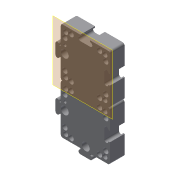
# Autodesk Inventor part: 30_cellSTORM_UC2_motorized_xystage_coupler_fiberlauncher
Saved by Autodesk Inventor 2022 (Build 260153000, 153)
## iProperties
Created: 2021-10-28
Part Number: 30_cellSTORM_UC2_motorized_xystage_coupler_fiberlauncher
Material: Generic
Document SubType Name: Modeling
Designer: diederichbenedict
Density: 1 g/cm^3
Appearance: Default
Author: diederichbenedict
Autodesk Inventor part; units mm, degrees
ref_plane "YZ Plane" through (0, 0, 0) normal (1, 0, 0) x (0, 1, 0)
ref_plane "XZ Plane" through (0, 0, 0) normal (0, 1, 0) x (-1, 0, 0)
ref_plane "XY Plane" through (0, 0, 0) normal (0, 0, 1) x (1, 0, 0)
ref_plane "Work Plane1" through (0, 100, 0) normal (0, 0, 1) x (1, 0, 0)
sketch "Sketch1" plane through (0, 100, 0) normal (0, 0, 1) x (1, 0, 0)
  circle A0 centre (-5.5948, 23.1279) radius 1.5 projected
  line L0 (30.2052, 32.2052) -> (0.2052, 32.2052) projected
  arc A1 (32.2052, 30.2052) -> (30.2052, 32.2052) centre (30.2052, 30.2052) ccw projected
  line L1 (32.2052, 30.2052) -> (32.2052, 0.2052) projected
  arc A2 (30.2052, -1.7948) -> (32.2052, 0.2052) centre (30.2052, 0.2052) ccw projected
  line L2 (15.6052, -1.7948) -> (30.2052, -1.7948) projected
  circle A3 centre (15.6052, -5.7948) radius 4 projected
  line L3 (0.2052, -1.7948) -> (15.6052, -1.7948) projected
  arc A4 (-1.7948, 0.2052) -> (0.2052, -1.7948) centre (0.2052, 0.2052) ccw projected
  line L4 (-1.7948, 0.2052) -> (-1.7948, 15.4052) projected
  circle A5 centre (-5.7948, 15.4052) radius 4 projected
  line L5 (-1.7948, 15.4052) -> (-1.7948, 30.2052) projected
  arc A6 (0.2052, 32.2052) -> (-1.7948, 30.2052) centre (0.2052, 30.2052) ccw projected
  circle A7 centre (-4.7948, -4.7948) radius 2.425 projected
  circle A8 centre (0.7052, -5.5948) radius 2.65 projected
  circle A9 centre (-5.5948, 0.7052) radius 2.65 projected
  circle A10 centre (-5.5948, 29.7052) radius 2.65 projected
  circle A11 centre (0.7052, 36.0052) radius 2.65 projected
  circle A12 centre (-4.7948, 35.2052) radius 2.425 projected
  circle A13 centre (36.0052, 0.7052) radius 2.65 projected
  circle A14 centre (29.7052, -5.5948) radius 2.65 projected
  circle A15 centre (35.2052, -4.7948) radius 2.425 projected
  circle A16 centre (36.0052, 29.7052) radius 2.65 projected
  circle A17 centre (29.7052, 36.0052) radius 2.65 projected
  circle A18 centre (35.2052, 35.2052) radius 2.425 projected
  line L6 (20.0856, 40.2052) -> (20.0856, 39.0762) projected
  arc A19 (20.0856, 39.0762) -> (20.4256, 38.6775) centre (20.4974, 39.083) ccw projected
  line L7 (20.4256, 38.6775) -> (20.5462, 38.647) projected
  arc A20 (20.0038, 34.5391) -> (20.5462, 38.647) centre (20.2052, 36.6023) ccw projected
  line L8 (20.0038, 34.5391) -> (10.2052, 34.5391) projected
  arc A21 (9.7873, 38.6768) -> (10.2052, 34.5391) centre (10.2052, 36.6291) ccw projected
  arc A22 (9.7873, 38.6768) -> (10.1151, 39.0783) centre (9.7054, 39.0783) ccw projected
  line L9 (10.1151, 39.0783) -> (10.1151, 40.2052) projected
  line L10 (10.1151, 40.2052) -> (-7.7948, 40.2052) projected
  arc A23 (-7.7948, 40.2052) -> (-9.7948, 38.2052) centre (-7.7948, 38.2052) ccw projected
  line L11 (-9.7948, 20.2052) -> (-9.7948, 38.2052) projected
  line L12 (-10.8453, 20.2052) -> (-9.7948, 20.2052) projected
  arc A24 (-11.3352, 20.6052) -> (-10.8453, 20.2052) centre (-10.8453, 20.7052) ccw projected
  arc A25 (-11.3352, 20.6052) -> (-15.2948, 20.2052) centre (-13.2948, 20.2052) ccw projected
  line L13 (-15.2948, 10.2052) -> (-15.2948, 20.2052) projected
  arc A26 (-15.2948, 10.2052) -> (-11.3352, 9.8052) centre (-13.2948, 10.2052) ccw projected
  arc A27 (-10.8453, 10.2052) -> (-11.3352, 9.8052) centre (-10.8453, 9.7052) ccw projected
  line L14 (-9.7948, 10.2052) -> (-10.8453, 10.2052) projected
  line L15 (-9.7948, -7.7948) -> (-9.7948, 10.2052) projected
  arc A28 (-9.7948, -7.7948) -> (-7.7948, -9.7948) centre (-7.7948, -7.7948) ccw projected
  line L16 (-7.7948, -9.7948) -> (10.2052, -9.7948) projected
  line L17 (10.2052, -10.8453) -> (10.2052, -9.7948) projected
  arc A29 (9.8052, -11.3352) -> (10.2052, -10.8453) centre (9.7052, -10.8453) ccw projected
  arc A30 (9.8052, -11.3352) -> (10.2052, -15.2948) centre (10.2052, -13.2948) ccw projected
  line L18 (20.2052, -15.2948) -> (10.2052, -15.2948) projected
  arc A31 (20.2052, -15.2948) -> (20.6052, -11.3352) centre (20.2052, -13.2948) ccw projected
  arc A32 (20.2052, -10.8453) -> (20.6052, -11.3352) centre (20.7052, -10.8453) ccw projected
  line L19 (20.2052, -9.7948) -> (20.2052, -10.8453) projected
  line L20 (20.2052, -9.7948) -> (38.2052, -9.7948) projected
  arc A33 (38.2052, -9.7948) -> (40.2052, -7.7948) centre (38.2052, -7.7948) ccw projected
  line L21 (40.2052, 10.3249) -> (40.2052, -7.7948) projected
  line L22 (40.2052, 10.3249) -> (39.0762, 10.3249) projected
  arc A34 (39.0762, 10.3249) -> (38.6775, 9.9849) centre (39.083, 9.9131) ccw projected
  line L23 (38.6775, 9.9849) -> (38.647, 9.8643) projected
  arc A35 (34.5391, 10.4067) -> (38.647, 9.8643) centre (36.6023, 10.2052) ccw projected
  line L24 (34.5391, 10.4067) -> (34.5391, 20.2052) projected
  arc A36 (38.6768, 20.6232) -> (34.5391, 20.2052) centre (36.6291, 20.2052) ccw projected
  arc A37 (38.6768, 20.6232) -> (39.0783, 20.2953) centre (39.0783, 20.7051) ccw projected
  line L25 (39.0783, 20.2953) -> (40.2052, 20.2953) projected
  line L26 (40.2052, 38.2052) -> (40.2052, 20.2953) projected
  arc A38 (40.2052, 38.2052) -> (38.2052, 40.2052) centre (38.2052, 38.2052) ccw projected
  line L27 (38.2052, 40.2052) -> (20.0856, 40.2052) projected
  circle A39 centre (-5.5948, -26.8721) radius 1.5 projected
  line L28 (30.2052, -17.7948) -> (0.2052, -17.7948) projected
  arc A40 (32.2052, -19.7948) -> (30.2052, -17.7948) centre (30.2052, -19.7948) ccw projected
  line L29 (32.2052, -19.7948) -> (32.2052, -49.7948) projected
  arc A41 (30.2052, -51.7948) -> (32.2052, -49.7948) centre (30.2052, -49.7948) ccw projected
  line L30 (15.6052, -51.7948) -> (30.2052, -51.7948) projected
  circle A42 centre (15.6052, -55.7948) radius 4 projected
  line L31 (0.2052, -51.7948) -> (15.6052, -51.7948) projected
  arc A43 (-1.7948, -49.7948) -> (0.2052, -51.7948) centre (0.2052, -49.7948) ccw projected
  line L32 (-1.7948, -49.7948) -> (-1.7948, -34.5948) projected
  circle A44 centre (-5.7948, -34.5948) radius 4 projected
  line L33 (-1.7948, -34.5948) -> (-1.7948, -19.7948) projected
  arc A45 (0.2052, -17.7948) -> (-1.7948, -19.7948) centre (0.2052, -19.7948) ccw projected
  circle A46 centre (-4.7948, -54.7948) radius 2.425 projected
  circle A47 centre (0.7052, -55.5948) radius 2.65 projected
  circle A48 centre (-5.5948, -49.2948) radius 2.65 projected
  circle A49 centre (-5.5948, -20.2948) radius 2.65 projected
  circle A50 centre (0.7052, -13.9948) radius 2.65 projected
  circle A51 centre (-4.7948, -14.7948) radius 2.425 projected
  circle A52 centre (36.0052, -49.2948) radius 2.65 projected
  circle A53 centre (29.7052, -55.5948) radius 2.65 projected
  circle A54 centre (35.2052, -54.7948) radius 2.425 projected
  circle A55 centre (36.0052, -20.2948) radius 2.65 projected
  circle A56 centre (29.7052, -13.9948) radius 2.65 projected
  circle A57 centre (35.2052, -14.7948) radius 2.425 projected
  line L34 (20.0856, -9.7948) -> (20.0856, -10.9238) projected
  arc A58 (20.0856, -10.9238) -> (20.4256, -11.3225) centre (20.4974, -10.917) ccw projected
  line L35 (20.4256, -11.3225) -> (20.5462, -11.353) projected
  arc A59 (20.0038, -15.4609) -> (20.5462, -11.353) centre (20.2052, -13.3977) ccw projected
  line L36 (20.0038, -15.4609) -> (10.2052, -15.4609) projected
  arc A60 (9.7873, -11.3232) -> (10.2052, -15.4609) centre (10.2052, -13.3709) ccw projected
  arc A61 (9.7873, -11.3232) -> (10.1151, -10.9217) centre (9.7054, -10.9217) ccw projected
  line L37 (10.1151, -10.9217) -> (10.1151, -9.7948) projected
  line L38 (10.1151, -9.7948) -> (-7.7948, -9.7948) projected
  arc A62 (-7.7948, -9.7948) -> (-9.7948, -11.7948) centre (-7.7948, -11.7948) ccw projected
  line L39 (-9.7948, -29.7948) -> (-9.7948, -11.7948) projected
  line L40 (-10.8453, -29.7948) -> (-9.7948, -29.7948) projected
  arc A63 (-11.3352, -29.3948) -> (-10.8453, -29.7948) centre (-10.8453, -29.2948) ccw projected
  arc A64 (-11.3352, -29.3948) -> (-15.2948, -29.7948) centre (-13.2948, -29.7948) ccw projected
  line L41 (-15.2948, -39.7948) -> (-15.2948, -29.7948) projected
  arc A65 (-15.2948, -39.7948) -> (-11.3352, -40.1948) centre (-13.2948, -39.7948) ccw projected
  arc A66 (-10.8453, -39.7948) -> (-11.3352, -40.1948) centre (-10.8453, -40.2948) ccw projected
  line L42 (-9.7948, -39.7948) -> (-10.8453, -39.7948) projected
  line L43 (-9.7948, -57.7948) -> (-9.7948, -39.7948) projected
  arc A67 (-9.7948, -57.7948) -> (-7.7948, -59.7948) centre (-7.7948, -57.7948) ccw projected
  line L44 (-7.7948, -59.7948) -> (10.2052, -59.7948) projected
  line L45 (10.2052, -60.8453) -> (10.2052, -59.7948) projected
  arc A68 (9.8052, -61.3352) -> (10.2052, -60.8453) centre (9.7052, -60.8453) ccw projected
  arc A69 (9.8052, -61.3352) -> (10.2052, -65.2948) centre (10.2052, -63.2948) ccw projected
  line L46 (20.2052, -65.2948) -> (10.2052, -65.2948) projected
  arc A70 (20.2052, -65.2948) -> (20.6052, -61.3352) centre (20.2052, -63.2948) ccw projected
  arc A71 (20.2052, -60.8453) -> (20.6052, -61.3352) centre (20.7052, -60.8453) ccw projected
  line L47 (20.2052, -59.7948) -> (20.2052, -60.8453) projected
  line L48 (20.2052, -59.7948) -> (38.2052, -59.7948) projected
  arc A72 (38.2052, -59.7948) -> (40.2052, -57.7948) centre (38.2052, -57.7948) ccw projected
  line L49 (40.2052, -39.6751) -> (40.2052, -57.7948) projected
  line L50 (40.2052, -39.6751) -> (39.0762, -39.6751) projected
  arc A73 (39.0762, -39.6751) -> (38.6775, -40.0151) centre (39.083, -40.0869) ccw projected
  line L51 (38.6775, -40.0151) -> (38.647, -40.1357) projected
  arc A74 (34.5391, -39.5933) -> (38.647, -40.1357) centre (36.6023, -39.7948) ccw projected
  line L52 (34.5391, -39.5933) -> (34.5391, -29.7948) projected
  arc A75 (38.6768, -29.3768) -> (34.5391, -29.7948) centre (36.6291, -29.7948) ccw projected
  arc A76 (38.6768, -29.3768) -> (39.0783, -29.7047) centre (39.0783, -29.2949) ccw projected
  line L53 (39.0783, -29.7047) -> (40.2052, -29.7047) projected
  line L54 (40.2052, -11.7948) -> (40.2052, -29.7047) projected
  arc A77 (40.2052, -11.7948) -> (38.2052, -9.7948) centre (38.2052, -11.7948) ccw projected
  line L55 (38.2052, -9.7948) -> (20.0856, -9.7948) projected
  point P0 (0, -100)
  point P1 (21.6421, -11.9035)
  constraints: 2 horizontal alignment, 2 vertical alignment
extrude "Extrusion1" add sketch "Sketch1" against normal blind 12 contours A1 L1 A2 L2 L3 A4 L4 L5 A6 L0 | A3 | L27 A38 L26 L25 A37 A36 L24 A35 L23 A34 L22 L21 A33 L20 L55 L34 A58 L35 A59 A31 L18 A30 A29 L17 L16 A28 L15 L14 A27 A26 L13 A25 A24 L12 L11 A23 L10 L9 A22 A21 L8 A20 L7 A19 L6 | A77 L54 L53 A76 A75 L52 A74 L51 A73 L50 L49 A72 L48 L47 A71 A70 L46 A69 A68 L45 L44 A67 L43 L42 A66 A65 L41 A64 A63 L40 L39 A62 L16 L37 A61 A60 L36 A59 A31 A32 L19 L20 | L19 A32 A31 A59 L35 A58 L34 L55 | A59 L36 A60 A61 L37 L16 L17 A29 A30 L18 A31 | A40 L29 A41 L30 L31 A43 L32 L33 A45 L28
sketch "Sketch2" plane through (0, 100, -12) normal (0, 0, -1) x (-1, 0, 0)
  line L0 (-40.2052, 10.3249) -> (-40.2052, -7.7948) projected
  arc A0 (-40.2052, -7.7948) -> (-38.2052, -9.7948) centre (-38.2052, -7.7948) ccw projected
  arc A1 (-38.2052, -9.7948) -> (-40.2052, -11.7948) centre (-38.2052, -11.7948) ccw projected
  line L1 (-40.2052, -11.7948) -> (-40.2052, -29.7047) projected
  line L2 (-40.2052, -29.7047) -> (-39.0783, -29.7047) projected
  arc A2 (-39.0783, -29.7047) -> (-38.6768, -29.3768) centre (-39.0783, -29.2949) ccw projected
  arc A3 (-34.5391, -29.7948) -> (-38.6768, -29.3768) centre (-36.6291, -29.7948) ccw projected
  line L3 (-34.5391, -29.7948) -> (-34.5391, -39.5933) projected
  arc A4 (-38.647, -40.1357) -> (-34.5391, -39.5933) centre (-36.6023, -39.7948) ccw projected
  line L4 (-38.647, -40.1357) -> (-38.6775, -40.0151) projected
  arc A5 (-38.6775, -40.0151) -> (-39.0762, -39.6751) centre (-39.083, -40.0869) ccw projected
  line L5 (-39.0762, -39.6751) -> (-40.2052, -39.6751) projected
  line L6 (-40.2052, -39.6751) -> (-40.2052, -57.7948) projected
  arc A6 (-40.2052, -57.7948) -> (-38.2052, -59.7948) centre (-38.2052, -57.7948) ccw projected
  line L7 (-38.2052, -59.7948) -> (-20.2052, -59.7948) projected
  line L8 (-20.2052, -59.7948) -> (-20.2052, -60.8453) projected
  arc A7 (-20.6052, -61.3352) -> (-20.2052, -60.8453) centre (-20.7052, -60.8453) ccw projected
  arc A8 (-20.6052, -61.3352) -> (-20.2052, -65.2948) centre (-20.2052, -63.2948) ccw projected
  line L9 (-20.2052, -65.2948) -> (-10.2052, -65.2948) projected
  arc A9 (-10.2052, -65.2948) -> (-9.8052, -61.3352) centre (-10.2052, -63.2948) ccw projected
  arc A10 (-10.2052, -60.8453) -> (-9.8052, -61.3352) centre (-9.7052, -60.8453) ccw projected
  line L10 (-10.2052, -60.8453) -> (-10.2052, -59.7948) projected
  line L11 (-10.2052, -59.7948) -> (7.7948, -59.7948) projected
  arc A11 (7.7948, -59.7948) -> (9.7948, -57.7948) centre (7.7948, -57.7948) ccw projected
  line L12 (9.7948, -57.7948) -> (9.7948, -39.7948) projected
  line L13 (9.7948, -39.7948) -> (10.8453, -39.7948) projected
  arc A12 (11.3352, -40.1948) -> (10.8453, -39.7948) centre (10.8453, -40.2948) ccw projected
  arc A13 (11.3352, -40.1948) -> (15.2948, -39.7948) centre (13.2948, -39.7948) ccw projected
  line L14 (15.2948, -39.7948) -> (15.2948, -29.7948) projected
  arc A14 (15.2948, -29.7948) -> (11.3352, -29.3948) centre (13.2948, -29.7948) ccw projected
  arc A15 (10.8453, -29.7948) -> (11.3352, -29.3948) centre (10.8453, -29.2948) ccw projected
  line L15 (10.8453, -29.7948) -> (9.7948, -29.7948) projected
  line L16 (9.7948, -29.7948) -> (9.7948, -11.7948) projected
  arc A16 (9.7948, -11.7948) -> (7.7948, -9.7948) centre (7.7948, -11.7948) ccw projected
  arc A17 (7.7948, -9.7948) -> (9.7948, -7.7948) centre (7.7948, -7.7948) ccw projected
  line L17 (9.7948, -7.7948) -> (9.7948, 10.2052) projected
  line L18 (9.7948, 10.2052) -> (10.8453, 10.2052) projected
  arc A18 (11.3352, 9.8052) -> (10.8453, 10.2052) centre (10.8453, 9.7052) ccw projected
  arc A19 (11.3352, 9.8052) -> (15.2948, 10.2052) centre (13.2948, 10.2052) ccw projected
  line L19 (15.2948, 10.2052) -> (15.2948, 20.2052) projected
  arc A20 (15.2948, 20.2052) -> (11.3352, 20.6052) centre (13.2948, 20.2052) ccw projected
  arc A21 (10.8453, 20.2052) -> (11.3352, 20.6052) centre (10.8453, 20.7052) ccw projected
  line L20 (10.8453, 20.2052) -> (9.7948, 20.2052) projected
  line L21 (9.7948, 20.2052) -> (9.7948, 38.2052) projected
  arc A22 (9.7948, 38.2052) -> (7.7948, 40.2052) centre (7.7948, 38.2052) ccw projected
  line L22 (7.7948, 40.2052) -> (-10.1151, 40.2052) projected
  line L23 (-10.1151, 40.2052) -> (-10.1151, 39.0783) projected
  arc A23 (-10.1151, 39.0783) -> (-9.7873, 38.6768) centre (-9.7054, 39.0783) ccw projected
  arc A24 (-10.2052, 34.5391) -> (-9.7873, 38.6768) centre (-10.2052, 36.6291) ccw projected
  line L24 (-10.2052, 34.5391) -> (-20.0038, 34.5391) projected
  arc A25 (-20.5462, 38.647) -> (-20.0038, 34.5391) centre (-20.2052, 36.6023) ccw projected
  line L25 (-20.5462, 38.647) -> (-20.4256, 38.6775) projected
  arc A26 (-20.4256, 38.6775) -> (-20.0856, 39.0762) centre (-20.4974, 39.083) ccw projected
  line L26 (-20.0856, 39.0762) -> (-20.0856, 40.2052) projected
  line L27 (-20.0856, 40.2052) -> (-38.2052, 40.2052) projected
  arc A27 (-38.2052, 40.2052) -> (-40.2052, 38.2052) centre (-38.2052, 38.2052) ccw projected
  line L28 (-40.2052, 38.2052) -> (-40.2052, 20.2953) projected
  line L29 (-40.2052, 20.2953) -> (-39.0783, 20.2953) projected
  arc A28 (-39.0783, 20.2953) -> (-38.6768, 20.6232) centre (-39.0783, 20.7051) ccw projected
  arc A29 (-34.5391, 20.2052) -> (-38.6768, 20.6232) centre (-36.6291, 20.2052) ccw projected
  line L30 (-34.5391, 20.2052) -> (-34.5391, 10.4067) projected
  arc A30 (-38.647, 9.8643) -> (-34.5391, 10.4067) centre (-36.6023, 10.2052) ccw projected
  line L31 (-38.647, 9.8643) -> (-38.6775, 9.9849) projected
  arc A31 (-38.6775, 9.9849) -> (-39.0762, 10.3249) centre (-39.083, 9.9131) ccw projected
  line L32 (-39.0762, 10.3249) -> (-40.2052, 10.3249) projected
  circle A32 centre (-29.7052, 36.0052) radius 2.65 projected
  circle A33 centre (-35.2052, -4.7948) radius 2.425 projected
  circle A34 centre (-36.0052, 0.7052) radius 2.65 projected
  circle A35 centre (5.7948, 15.4052) radius 4 projected
  circle A36 centre (5.5948, 23.1279) radius 1.5 projected
  circle A37 centre (4.7948, -4.7948) radius 2.425 projected
  circle A38 centre (-0.7052, -5.5948) radius 2.65 projected
  circle A39 centre (5.5948, 0.7052) radius 2.65 projected
  circle A40 centre (5.5948, 29.7052) radius 2.65 projected
  circle A41 centre (-0.7052, 36.0052) radius 2.65 projected
  circle A42 centre (4.7948, 35.2052) radius 2.425 projected
  circle A43 centre (-29.7052, -5.5948) radius 2.65 projected
  circle A44 centre (-36.0052, 29.7052) radius 2.65 projected
  circle A45 centre (-35.2052, 35.2052) radius 2.425 projected
  circle A46 centre (-15.6052, -55.7948) radius 4 projected
  circle A47 centre (-35.2052, -14.7948) radius 2.425 projected
  circle A48 centre (-36.0052, -20.2948) radius 2.65 projected
  circle A49 centre (-29.7052, -55.5948) radius 2.65 projected
  circle A50 centre (4.7948, -14.7948) radius 2.425 projected
  circle A51 centre (5.5948, -20.2948) radius 2.65 projected
  circle A52 centre (-0.7052, -55.5948) radius 2.65 projected
  circle A53 centre (5.7948, -34.5948) radius 4 projected
  circle A54 centre (5.5948, -26.8721) radius 1.5 projected
  circle A55 centre (4.7948, -54.7948) radius 2.425 projected
  circle A56 centre (5.5948, -49.2948) radius 2.65 projected
  circle A57 centre (-0.7052, -13.9948) radius 2.65 projected
  circle A58 centre (-36.0052, -49.2948) radius 2.65 projected
  circle A59 centre (-35.2052, -54.7948) radius 2.425 projected
  circle A60 centre (-29.7052, -13.9948) radius 2.65 projected
  line L33 (-6.922, 6.881) -> (-26.922, 18.428)
  line L34 (-26.922, 18.428) -> (-6.922, 29.975)
  line L35 (-6.922, 29.975) -> (-6.922, 6.881)
  line L36 (9.7948, 20.2052) -> (9.7948, 38.2052) projected
  point P0 (0, -100)
  point P1 (-13.5887, 18.428)
  dimension "d2" = 20
  constraints: 6 end point, 1 parallel, 7 other
  measures "d2" distance from line of L33.end L35
hole "Hole1" at (26.922, 118.428, -12) at (6.922, 106.881, -12) at (6.922, 129.975, -12) direction (0, 0, 1) diameter 2.8 end through all
pattern_linear "Rectangular Pattern1" count 5 spacing 10 along (0, -1, 0) of "Hole1"
body "Solid1"
